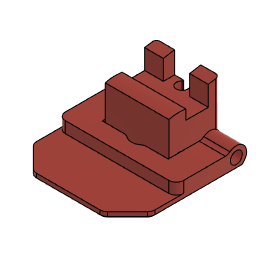
Simplish-Hinge-v0.1 v7 (Autodesk Fusion 360 design; units mm, degrees)
Autodesk Fusion 360 part; units mm, degrees
note: some values were not read from the file. Chosen so that the rebuilt part matches the saved one: a direction; a side; where a step starts. Set by a fixed rule: which sketch regions a step uses.
sketch "Sketch1" plane through (0, 0, 0) normal (0, 0, 1) x (1, 0, 0)
  line L0 (0, 0) -> (0, 13.5)
  line L1 (0, 13.5) -> (9.2274, 13.5)
  line L2 (10.8, 12) -> (10.8, 1.6488)
  line L3 (9.2274, 0) -> (0, 0)
  line L4 (0, 13.5) -> (-5.8, 13.5)
  line L5 (-5.8, 13.5) -> (-5.3, 10.5)
  line L6 (-5.3, 10.5) -> (0, 10.5)
  circle A0 centre (8.05, 2.75) radius 2.75
  circle A1 centre (8.05, 2.75) radius 1.6
  line L7 (9.2274, 0) -> (10.8, 1.6488)
  line L8 (5.9287, 4.5) -> (-8, 4.5)
  line L9 (-8, 4.5) -> (-8, 1.5)
  line L10 (-8, 1.5) -> (-21, 1.5)
  line L11 (-21, 1.5) -> (-21, 0)
  line L12 (-21, 0) -> (0, 0)
  line L13 (-4.3, 13.5) -> (-4.3, 10.5)
  line L14 (0, 10.5) -> (7.7, 10.5)
  line L15 (7.7, 10.5) -> (7.7, 13.5)
  line L16 (7.7, 9.25) -> (10.7, 9.25) construction
  line L17 (10.7, 9.25) -> (10.7, 14.75) construction
  line L18 (10.7, 14.75) -> (7.7, 14.75) construction
  line L19 (7.7, 14.75) -> (7.7, 9.25) construction
  line L20 (0, 13.5) -> (7.9, 13.5) construction
  line L21 (7.9, 13.5) -> (7.9, 20.5) construction
  line L22 (7.9, 20.5) -> (0, 20.5) construction
  line L23 (0, 20.5) -> (0, 13.5) construction
  line L24 (5.3, 2.75) -> (5.3, 31.8) construction
  line L25 (5.3, 31.8) -> (6.8, 31.8) construction
  line L26 (6.8, 31.8) -> (6.8, 18.8) construction
  line L27 (6.8, 18.8) -> (9.8, 18.8) construction
  line L28 (9.8, 18.8) -> (9.8, 4.8713) construction
  line L29 (9.8, 19.8) -> (7.8, 19.8) construction
  line L30 (7.8, 19.8) -> (7.8, 31.8) construction
  line L31 (7.8, 31.8) -> (9.8, 31.8) construction
  line L32 (9.8, 31.8) -> (9.8, 19.8) construction
  line L33 (6.5, 20.5) -> (7.9, 19.1) construction
  arc A2 (-3.1281, 4.5) -> (-2.925, 0) centre (8.05, 2.75) ccw
  line L34 (9.2274, 13.5) -> (10.8, 12)
  circle A3 centre (8.05, 2.75) radius 10.8143
  dimension "d1" = 8
  dimension "d2" = 13
  dimension "d3" = 9
  dimension "d4" = 3
  dimension "d5" = 5.3
  dimension "d6" = 0.5
  dimension "d7" = 5.5
  dimension "d8" = 3.2
  dimension "d9" = 1
  dimension "d10" = 12
  dimension "d11" = 5.5
  dimension "d12" = 3
  dimension "d13" = 3
  dimension "d14" = 1.5
  dimension "d16" = 7
  dimension "d18" = 1
  dimension "d19" = 1
  dimension "d21" = 7.9
  dimension "d22" = 1.4
  dimension "d51" = 0.1
  dimension "d64" = 1.5
  dimension "d97" = 0.5
  constraint coincident L0.start L3.end
  constraint vertical L0
  constraint perpendicular L0 L1
  constraint perpendicular L1 L2
  constraint perpendicular L0 L3
  constraint perpendicular L0 L4
  constraint coincident L0 L6.end
  constraint perpendicular L0 L6
  constraint concentric A0 A1
  constraint coincident A0 L8.start
  constraint parallel L3 L8
  constraint perpendicular L8 L9
  constraint perpendicular L9 L10
  constraint perpendicular L8 L11
  constraint perpendicular L0 L12
  constraint tangent A0 L7
  constraint tangent L2 A0
  constraint tangent L3 A0
  constraint coincident L4 L13.start
  constraint coincident L6 L13.end
  constraint perpendicular L6 L13
  constraint perpendicular L0 L14
  constraint coincident L1 L15.end
  constraint perpendicular L1 L15
  constraint horizontal L16
  constraint vertical L17
  constraint horizontal L18
  constraint vertical L19
  constraint midpoint L15 L19
  constraint horizontal L20
  constraint vertical L21
  constraint horizontal L22
  constraint vertical L23
  constraint coincident A0 L24.start
  constraint tangent A0 L24
  constraint perpendicular L22 L24
  constraint perpendicular L24 L25
  constraint perpendicular L22 L26
  constraint perpendicular L26 L27
  constraint coincident A0 L28.end
  constraint perpendicular L27 L28
  constraint horizontal L29
  constraint vertical L30
  constraint horizontal L31
  constraint vertical L32
  constraint equal L9 L27
  constraint equal L11 L25
  constraint equal L10 L26
  constraint equal L8 L28
  constraint vertical L27.end L29.start
  constraint horizontal L25.end L31.end
  constraint coincident L22 L33.start
  constraint coincident L21 L33.end
  constraint coincident L12 A2.end
  constraint coincident L8 A2.start
  constraint perpendicular L7 L34
  constraint vertical L3.start L1.end
  constraint coincident L1.end A3
  constraint coincident A0.centre A1.centre
  measures "d1" distance of L0 L8.end
  measures "d2" distance of L9.end L10.end
  measures "d3" distance of L1 L8
  measures "d4" distance of L4 L6
  measures "d5" distance of L5.end L6.end
  measures "d6" horizontal distance of L4.end L5.end
  measures "d7" diameter of A0
  measures "d8" diameter of A1
  measures "d9" distance of L5.end L13
  measures "d10" distance of L13.end L14.end
  measures "d11" distance of L16.end L17.end
  measures "d12" distance of L17.end L18.end
  measures "d13" distance of L8.end L9.end
  measures "d14" distance of L10.end L11.end
  measures "d16" distance of L0.end L22.end
  measures "d18" distance of L25.end L30.end
  measures "d19" distance of L27.end L29.start
  measures "d21" distance of L21.end L22.end
  measures "d22" distance of L21.end L33.start
  measures "d51" distance of L21 L30
  measures "d64" distance of L1 L2.start
  measures "d97" distance of A2 A3
extrude "Extrude5" add sketch "Sketch1" along normal blind 31.6 contours L0 L3 A0 L8 | L0 L8 L12 A3 | L8 L12 A2 A3 | A0 | L8 L9 L10 L11 L12 A2 | L3 A0 L7 makes body 1
extrude "Extrude6" cut sketch "Sketch1" along normal blind 17.6 from surface at 7 contours L0 L3 A0 L8 | L0 L8 L12 A3 | L8 L12 A2 A3 | A0 | L3 A0 L7 bodies 1
extrude "Extrude7" add sketch "Sketch1" along normal up to surface (17 mm away) from surface at 7.3 separate body contours L0 L4 L6 L13 | L0 L14 A3 | L0 L1 L14 A3 | L0 L1 L2 A0 L8 L14 L15 L34 A3 | L4 L5 L6 L13 | L1 L14 L15 A3 | L0 L3 A0 L8 | L0 L8 L12 A3 | A0 | L2 A0 L7 makes body 2
extrude "Extrude8" cut sketch "Sketch1" along normal up to surface (7 mm away) from surface at 12.3 contours L0 L4 L6 L13 | L4 L5 L6 L13 bodies 2
sketch "Sketch3" plane through (0, 0, 0) normal (-1, 0, 0) x (0, -1, 0)
  line L0 (-4.5, 24.3) -> (-10.5, 24.3)
  line L1 (-10.5, 24.3) -> (-10.5, 19.3)
  line L2 (-10.5, 19.3) -> (-13.5, 19.3)
  line L3 (-13.5, 19.3) -> (-13.5, 12.3)
  line L4 (-13.5, 12.3) -> (-10.5, 12.3)
  line L5 (-10.5, 12.3) -> (-10.5, 7.3)
  line L6 (-10.5, 7.3) -> (-4.5, 7.3)
  line L7 (-13.5, 15.8) -> (-10.5, 15.8) construction
  arc A0 (-13.5, 13.4951) -> (-13.5, 18.1049) centre (-12, 15.8) ccw
  arc A1 (-13.5, 15.4095) -> (-13.5, 16.1905) centre (-12, 15.8) ccw
  line L8 (-13.5, 18.1049) -> (-13.5, 13.4951)
  line L9 (-13.1, 18.3204) -> (-13.1, 13.2796)
  line L10 (-10.45, 18.0716) -> (-10.45, 13.5284)
  line L11 (-13.1, 14.25) -> (-10.45, 14.25)
  line L12 (-13.1, 17.35) -> (-10.45, 17.35)
  line L13 (-13.5, 16.892) -> (-13.1, 16.892)
  line L14 (-13.5, 14.708) -> (-13.1, 14.708)
  line L15 (-4.5, 7.3) -> (-4.5, 24.3)
  dimension "d65" = 3.1
  dimension "d66" = 5.5
  dimension "d67" = 0.4
  constraint midpoint L3 L7.start
  constraint perpendicular L1 L7
  constraint midpoint L7 A0.centre
  constraint concentric A0 A1
  constraint coincident L3 A0.end
  constraint coincident L3 A0.start
  constraint coincident L3 A1.end
  constraint coincident L3 A1.start
  constraint coincident A0 L9.start
  constraint coincident A0 L9.end
  constraint coincident A0 L10.start
  constraint coincident A0 L10.end
  constraint parallel L8 L10
  constraint coincident L10 L11.end
  constraint perpendicular L10 L11
  constraint coincident L9 L12.start
  constraint perpendicular L9 L12
  constraint coincident L9 L11.start
  constraint coincident L10 L12.end
  constraint vertical L1.end L7.end
  constraint tangent A1 L12
  constraint tangent A1 L10
  constraint tangent A1 L11
  constraint parallel L8 L9
  constraint coincident L8 L13.start
  constraint coincident L9 L13.end
  constraint coincident A1 L13.end
  constraint perpendicular L8 L13
  constraint symmetric L7 L13.start L14.start
  constraint symmetric L7 L13.end L14.end
  measures "d65" diameter of A1
  measures "d66" diameter of A0
  measures "d67" distance of L8 L9
extrude "Extrude9" cut sketch "Sketch3" against normal through all contours L3 A1 L8 L13 | L3 A1 L8 L9 | A1 L9 | L3 A1 L8 L14 bodies 2
extrude "Extrude10" cut sketch "Sketch3" against normal through all from surface at -6.5 contours L3 A0 L8 L9 L13 | L3 A1 L8 L13 | A0 L9 L10 L12 | L3 A0 L8 L9 L14 | L3 A1 L8 L9 | A1 L9 L12 | A0 L10 | L3 A1 L8 L14 | A0 L9 L10 L11 | A1 L10 L12 | A1 L9 L11 | A1 L10 L11 bodies 2
extrude "Extrude11" add sketch "Sketch3" against normal blind 0.2 from surface at -6.5 contours L3 A0 L8 L9 L13 | L3 A1 L8 L13 | A0 L9 L10 L12 | L3 A0 L8 L9 L14 | L3 A1 L8 L9 | A0 L10 | L3 A1 L8 L14 | A0 L9 L10 L11 bodies 2
extrude "Extrude12" add sketch "Sketch3" against normal blind 0.2 from surface at -6.7 contours L3 A0 L8 L9 L13 | L3 A1 L8 L13 | L3 A0 L8 L9 L14 | L3 A1 L8 L9 | A0 L10 | L3 A1 L8 L14 bodies 2
sketch "Sketch4" plane through (0, 1.5, 0) normal (0, 1, 0) x (-1, 0, 0)
  line L0 (8, 0) -> (21, 0)
  line L1 (21, 0) -> (21, 31.6)
  line L2 (21, 31.6) -> (8, 31.6)
  line L3 (8, 31.6) -> (8, 0)
  line L4 (14.5, 31.6) -> (21, 25.1)
  line L5 (14.5, 0) -> (21, 6.5)
  dimension "d78" = 45
  constraint midpoint L2 L4.start
  constraint coincident L1 L4.end
  constraint midpoint L0 L5.start
  constraint coincident L1 L5.end
  constraint perpendicular L4 L5
  measures "d78" angle of L2 L4
extrude "Extrude13" cut sketch "Sketch4" against normal through all contours L0 L1 L5 | L1 L2 L4 bodies 1
sketch "Sketch6" plane through (6.9, 0, 0) normal (1, 0, 0) x (0, 1, 0)
  arc A0 (10.45, 18.0716) -> (10.45, 13.5284) centre (12, 15.8) ccw
  line L0 (10.45, 13.5284) -> (10.45, 18.0716)
  circle A1 centre (12, 15.8) radius 3
  point P0 (12, 15.8)
  dimension "d90" = 6
  constraint coincident P0 A0.centre
  measures "d90" diameter of A1
ref_plane "WorkPlane1" through (2.5, 6.75, 15.8) normal (0, 0, 1) x (1, 0, 0)
sketch "Sketch7" plane through (2.5, 6.85, 15.8) normal (0, 0, 1) x (1, 0, 0)
  circle A0 centre (5.55, -4.1) radius 9.3212
  point P0 (4.4, 5.15)
  point P1 (5.55, -4.1)
  constraint coincident A0 P0
  constraint coincident A0.centre P1
sweep "Sweep1" cut profiles "Sketch6" path "Sketch7" along A0 section 1 contours A0 L0 | A1 bodies 1
fillet "Fillet1" radius 2 10 edges at (-14.5, 0.75, 31.6) (-21, 0.75, 25.1) (-8, 3, 31.6) (-21, 0.75, 6.5) (-14.5, 0.75, 0) (-8, 3, 0) (5.9287, 4.5, 28.1) (5.9287, 4.5, 3.5) (-3.2528, 2.2398, 18.031) (-3.2528, 2.2398, 13.569) on bodies 1
chamfer "Chamfer1" distance 0.4 angle 45 17 edges at (-2.2221, 0, 31.6) (-14.4369, 0, 31.4478) (-17.75, 0, 28.35) (-20.8478, 0, 25.0369) (-21, 0, 15.8) (-20.8478, 0, 6.5631) (-17.75, 0, 3.25) (-14.4369, 0, 0.1522) (-2.2221, 0, 0) (-2.925, 0, 21.6949) (-3.03, 0, 18.1595) (-3.9426, 0, 15.8005) (-3.03, 0, 13.4405) (-2.925, 0, 9.9051) (10.8, 6.8244, 24.3) (10.8, 6.8244, 7.3) (10.8, 9.25, 15.8) on bodies 1 2
fillet "Fillet2" radius 1 2 edges at (1.7137, 13.5, 24.3) (1.7137, 13.5, 7.3) on bodies 2
move_body "Align5" bodies 2 to x (0, 0, -1) y (0, 1, 0) z (1, 0, 0) at (-5, 0, 10.8)
move_body "Align6" bodies 1 to x (1, 0, 0) y (0, 0, 1) z (0, -1, 0) at (0, 0, 0)
move_body "Align7" bodies 1 to x (0, 1, 0) y (-1, 0, 0) z (0, 0, 1) at (-5.3, -28.3679, 0)
move_body "Move2" bodies 1 to x (1, 0, 0) y (0, 1, 0) z (0, 0, 1) at (0.3, 31, 0)
copy_body "Body->Comp3" bodies 1 removing the originals makes body 3 in component "Component"
copy_body "Body->Comp4" bodies 2 removing the originals makes body 4 in component "Component'"
component "Simplish-Hinge" placed x (1, 0, 0) y (0, 1, 0) z (0, 0, 1) at (0, 0, 0)
component "Component" placed x (1, 0, 0) y (0, 0, -1) z (0, 1, 0) at (0, 0, 13.4321) in component "Simplish-Hinge"
component "Component'" placed x (1, 0, 0) y (0, 1, 0) z (0, 0, 1) at (0, 0, 0) in component "Simplish-Hinge"
equation "d53 = 7 mm + 17.6 mm + 7 mm"
equation "d69 = -( 12 mm - 5.5 mm )"
